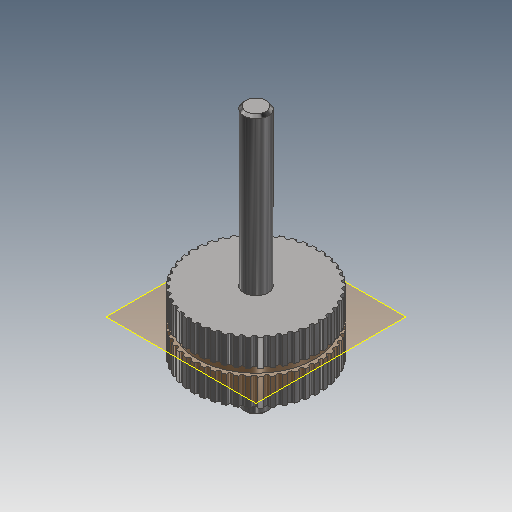
# Autodesk Inventor part: Nema 17 shaft
Saved by Autodesk Inventor 2020.2 (Build 242310000, 310)
## iProperties
Created: 2020-01-17
Part Number: Nema 17 shaft
Material: Stainless Steel
Document SubType Name: Modeling
Designer: james
Density: 8 g/cm^3
Appearance: Semi-Polished
Mass: 56.0374 g
Surface Area: 51.5245 cm^2
Volume: 7.00468 cm^3
Author: james
Autodesk Inventor part; units mm, degrees
ref_plane "YZ Plane" through (0, 0, 0) normal (1, 0, 0) x (0, 1, 0)
ref_plane "XZ Plane" through (0, 0, 0) normal (0, 1, 0) x (-1, 0, 0)
ref_plane "XY Plane" through (0, 0, 0) normal (0, 0, 1) x (1, 0, 0)
sketch "Sketch11" plane through (0, 0, 0) normal (0, 1, 0) x (-1, 0, 0)
  circle A0 centre (0, 0) radius 2.5
  dimension "d82" = 5
  constraints: 1 centre point, 1 coincident
  measures "d82" diameter of A0
extrude "Extrusion7" add sketch "Sketch11" along normal mid plane 53
chamfer "Chamfer1" distance 0.5 angle 45 2 edges at (2.5, 26.5, 0) (2.5, -26.5, 0)
sketch "Sketch12" plane through (0, 26.5, 0) normal (0, 1, 0) x (1, 0, 0)
  line L0 (1.5, 2) -> (-1.5, 2)
  line L1 (-1.5, 2) -> (-1.5, 2.5)
  line L2 (-1.5, 2.5) -> (1.5, 2.5)
  line L3 (1.5, 2.5) -> (1.5, 2)
  line L4 (1.5, 2) -> (-1.5, 2.5) construction
  line L5 (-1.5, 2) -> (1.5, 2.5) construction
  circle A0 centre (0, 0) radius 2.5 construction
  line L6 (0, 2) -> (0, -2.5) construction
  point P0 (0, 2.25)
  dimension "d88" = 4.5
  constraints: 14 end point, 3 midpoint, 2 parallel, 2 point on circle, 1 horizontal, 1 perpendicular, 1 tangent, 1 vertical
  measures "d88" distance of L6.start L6.end
extrude "Extrusion8" cut sketch "Sketch12" against normal blind 18
ref_plane "Work Plane6" through (0, -17.75, 0) normal (0, -1, 0) x (1, 0, 0)
sketch "Sketch13" plane through (0, -17.75, 0) normal (0, -1, 0) x (1, 0, 0)
  circle A0 centre (0, 0) radius 2.5 projected
  circle A1 centre (0, 0) radius 12.9
  dimension "d110" = 25.8
  constraints: 1 centre point, 1 coincident
  measures "d110" diameter of A1
extrude "Extrusion9" add sketch "Sketch13" against normal blind 5.5 separate body
ref_plane "Work Plane7" through (0, -10.75, 0) normal (0, 1, 0) x (1, 0, 0)
sketch "Sketch14" plane through (0, -10.75, 0) normal (0, 1, 0) x (1, 0, 0)
  circle A0 centre (0, 0) radius 12.9 projected
  circle A1 centre (0, 0) radius 2.5 projected
extrude "Extrusion10" add sketch "Sketch14" along normal blind 5.5 separate body
sketch "Sketch15" plane through (0, -5.25, 0) normal (0, 1, 0) x (1, 0, 0)
  circle A0 centre (0, 0) radius 12.9 projected
  circle A1 centre (0, 12.9) radius 0.5
  dimension "d97" = 1
  constraints: 2 vertical alignment, 1 centre point, 1 other
  measures "d97" diameter of A1
extrude "Extrusion11" cut sketch "Sketch15" against normal through all contours A1 A0 | A0 A1 picked at (0.0198, 12.7338) picked at (0.0186, 13.0649) bodies 3 2
pattern_circular "Circular Pattern1" count 45 over 360 about axis through (0, 0, 0) along (0, 1, 0) of "Extrusion11" bodies 2 3
sketch "Sketch16" plane through (0, -12.25, 0) normal (0, 1, 0) x (1, 0, 0)
  circle A0 centre (-0.0331, 0.051) radius 12
  circle A1 centre (0, 0) radius 2.5 projected
  dimension "d103" = 24
  constraints: 1 centre point
  measures "d103" diameter of A0
extrude "Extrusion12" add sketch "Sketch16" along normal up to surface (1.5 mm away) separate body
ref_plane "Work Plane8" through (0, -21.5, 0) normal (0, -1, 0) x (1, 0, 0)
sketch "Sketch17" plane through (0, -21.5, 0) normal (0, -1, 0) x (1, 0, 0)
  circle A0 centre (0, 0) radius 2.5 projected
  circle A1 centre (0, 0) radius 2
  dimension "d107" = 4
  constraints: 1 centre point
  measures "d107" diameter of A1
extrude "Extrusion13" cut sketch "Sketch17" against normal blind 0.75 bodies 1
body "Solid6"
body "Solid7"
body "Solid8"
body "Solid9"
